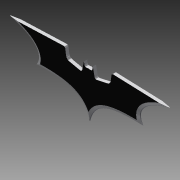
# Autodesk Inventor part: Batarang
Saved by Autodesk Inventor 2014 (Build 180170000, 170)
## iProperties
Created: 2013-12-21
Part Number: Batarang
Material: Generic
Document SubType Name: Modeling
Designer: william
Density: 1 g/cm^3
Appearance: Default
Author: william
Autodesk Inventor part; units mm, degrees
ref_plane "YZ Plane" through (0, 0, 0) normal (1, 0, 0) x (0, 1, 0)
ref_plane "XZ Plane" through (0, 0, 0) normal (0, 1, 0) x (-1, 0, 0)
ref_plane "XY Plane" through (0, 0, 0) normal (0, 0, 1) x (1, 0, 0)
sketch "Sketch1" plane through (0, 0, 0) normal (0, 0, 1) x (1, 0, 0)
  line L0 (-16.3551, -33.4322) -> (91.3246, -29.4519)
  line L1 (94.5837, -32.1667) -> (96.2868, -43.8498)
  line L2 (102.2167, -50.1985) -> (123.8401, -54.8738)
  arc A0 (94.5837, -32.1667) -> (91.3246, -29.4519) centre (91.4419, -32.6247) ccw
  arc A1 (96.2868, -43.8498) -> (102.2167, -50.1985) centre (103.8271, -42.7506) ccw
  line L3 (127.6144, -52.4415) -> (131.1971, -35.8715)
  line L4 (131.1971, -35.8715) -> (132.013, -41.4683)
  line L5 (135.6128, -44.1521) -> (139.8228, -43.5384)
  arc A2 (123.8401, -54.8738) -> (127.6144, -52.4415) centre (124.5111, -51.7705) ccw
  arc A3 (132.013, -41.4683) -> (135.6128, -44.1521) centre (135.1548, -41.0103) ccw
  line L6 (-16.3551, -33.4322) -> (32.8318, -47.0191) construction
  spline S0 degree 3 poles (-16.3551, -33.4322) (32.8318, -47.0191) (49.3977, -67.4844) (35.9265, -89.8885) knots 1 1 1 1 1.712271 1.712271 1.712271 1.712271
  line L7 (35.9265, -89.8885) -> (111.1968, -87.1062) construction
  line L8 (111.1968, -87.1062) -> (131.1971, -101.4022) construction
  line L9 (131.1971, -101.4022) -> (139.8228, -134.9505) construction
  spline S1 degree 3 poles (35.9265, -89.8885) (111.1968, -87.1062) (131.1971, -101.4022) (139.8228, -134.9505) knots 1 1 1 1 2 2 2 2
  line L10 (32.8318, -47.0191) -> (49.3977, -67.4844) construction
  line L11 (49.3977, -67.4844) -> (35.9265, -89.8885) construction
  line L12 (139.8228, -134.9505) -> (233.305, -134.9505) construction
  line L13 (296.0007, -33.4322) -> (188.3211, -29.4519)
  line L14 (185.062, -32.1667) -> (183.3589, -43.8498)
  line L15 (177.4289, -50.1985) -> (155.8056, -54.8738)
  arc A4 (188.3211, -29.4519) -> (185.062, -32.1667) centre (188.2038, -32.6247) ccw
  arc A5 (177.4289, -50.1985) -> (183.3589, -43.8498) centre (175.8186, -42.7506) ccw
  line L16 (152.0313, -52.4415) -> (148.4486, -35.8715)
  line L17 (148.4486, -35.8715) -> (147.6327, -41.4683)
  line L18 (144.0329, -44.1521) -> (139.8228, -43.5384)
  arc A6 (152.0313, -52.4415) -> (155.8056, -54.8738) centre (155.1346, -51.7705) ccw
  arc A7 (144.0329, -44.1521) -> (147.6327, -41.4683) centre (144.4909, -41.0103) ccw
  line L19 (296.0007, -33.4322) -> (246.8139, -47.0191) construction
  spline S2 degree 3 poles (296.0007, -33.4322) (246.8139, -47.0191) (230.2479, -67.4844) (243.7192, -89.8885) knots 1 1 1 1 1.712271 1.712271 1.712271 1.712271
  line L20 (243.7192, -89.8885) -> (168.4489, -87.1062) construction
  line L21 (168.4489, -87.1062) -> (148.4486, -101.4022) construction
  line L22 (148.4486, -101.4022) -> (139.8228, -134.9505) construction
  spline S3 degree 3 poles (243.7192, -89.8885) (168.4489, -87.1062) (148.4486, -101.4022) (139.8228, -134.9505) knots 1 1 1 1 2 2 2 2
  line L23 (246.8139, -47.0191) -> (230.2479, -67.4844) construction
  line L24 (230.2479, -67.4844) -> (243.7192, -89.8885) construction
  point P0 (0, 0)
  dimension "d1" = 3.175
  dimension "d2" = 7.62
  dimension "d4" = 3.175
  dimension "d5" = 3.175
  constraints: 26 end point, 16 point on circle, 8 centre point, 8 tangent, 2 parallel, 2 perpendicular, 1 horizontal, 12 other
  measures "d1" radius of A0
  measures "d2" radius of A1
  measures "d4" radius of A2
  measures "d5" radius of A3
extrude "Extrusion1" add sketch "Sketch1" along normal blind 6.35
chamfer "Chamfer1" distance 3.048 angle 45 8 edges at (166.7793, -98.7956, 6.35) (166.7793, -98.7956, 0) (112.8664, -98.7956, 6.35) (112.8664, -98.7956, 0) (33.2825, -58.3539, 6.35) (33.2825, -58.3539, 0) (246.3632, -58.3539, 6.35) (246.3632, -58.3539, 0)
chamfer "Chamfer2" distance 3.048 angle 45 8 edges at (169.1757, -94.4125, 0) (110.47, -94.4125, 0) (35.4048, -56.1557, 0) (244.2409, -56.1557, 0) (35.4048, -56.1557, 6.35) (110.47, -94.4125, 6.35) (169.1757, -94.4125, 6.35) (244.2409, -56.1557, 6.35)
body "Solid1"
